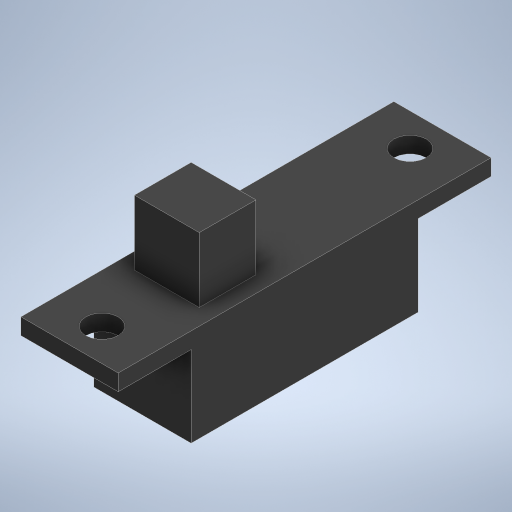
# Autodesk Inventor part: SlideSwitchj
Saved by Autodesk Inventor 2024.2 (Build 282272000, 272)
## iProperties
Created: 2024-05-04
Part Number: SlideSwitchj
Material: Generic
Document SubType Name: Modeling
Designer: ringl
Density: 1 g/cm^3
Appearance: Default(1)
Author: ringl
Autodesk Inventor part; units mm, degrees
ref_plane "YZ Plane" through (0, 0, 0) normal (1, 0, 0) x (0, 1, 0)
ref_plane "XZ Plane" through (0, 0, 0) normal (0, 1, 0) x (-1, 0, 0)
ref_plane "XY Plane" through (0, 0, 0) normal (0, 0, 1) x (1, 0, 0)
sketch "Sketch1" plane through (0, 0, 0) normal (0, 1, 0) x (-1, 0, 0)
  line L0 (0, 0) -> (6, 0)
  line L1 (6, 0) -> (6, -23)
  line L2 (6, -23) -> (0, -23)
  line L3 (0, -23) -> (0, 0)
  circle A0 centre (3, -2) radius 1
  circle A1 centre (3, -21) radius 1
  point P0 (3, 0)
  dimension "d0" = 6
  dimension "d1" = 23
  dimension "d2" = 2
  dimension "d3" = 2
  dimension "d4" = 19
  dimension "d5" = 2
  dimension "d6" = 3
  constraints: 8 end point, 2 centre point, 2 parallel, 1 horizontal, 1 midpoint, 1 perpendicular, 1 vertical alignment
  measures "d0" distance of L1.end L2.end
  measures "d1" distance of L0.end L1.end
  measures "d2" diameter of A0
  measures "d3" diameter of A1
  measures "d4" distance of A0.centre A1.centre
  measures "d5" distance of point (3, 0) A0.centre
  measures "d6" distance from line of L3 A1.centre
extrude "Extrusion1" add sketch "Sketch1" along normal blind 1
sketch "Sketch2" plane through (0, 0, 0) normal (0, -1, 0) x (1, 0, 0)
  line L0 (-6, -23) -> (-6, 0) projected
  line L1 (0, 0) -> (0, -23) projected
  line L2 (-6, -4.5) -> (0, -4.5)
  line L3 (0, -4.5) -> (0, -18.5)
  line L4 (0, -18.5) -> (-6, -18.5)
  line L5 (-6, -18.5) -> (-6, -4.5)
  line L6 (-6, 0) -> (0, 0) projected
  point P0 (-3, -18.5)
  dimension "d9" = 14
  dimension "d10" = 4.5
  constraints: 8 end point, 2 parallel, 2 point on line, 1 horizontal, 1 midpoint, 1 perpendicular
  measures "d9" distance from line of point (-3, -18.5) L2
  measures "d10" distance between parallel lines of L6 L2
extrude "Extrusion2" add sketch "Sketch2" along normal blind 5 contours L0 L2 L1 L4
sketch "Sketch3" plane through (0, 1, 0) normal (0, 1, 0) x (1, 0, 0)
  line L0 (-5, 6) -> (-1, 6)
  line L1 (-1, 6) -> (-1, 9.5)
  line L2 (-1, 9.5) -> (-5, 9.5)
  line L3 (-5, 9.5) -> (-5, 6)
  line L4 (-6, 23) -> (-6, 0) projected
  line L5 (-6, 0) -> (0, 0) projected
  dimension "d13" = 4
  dimension "d14" = 3.5
  dimension "d15" = 1
  dimension "d16" = 6
  constraints: 8 end point, 2 parallel, 1 horizontal, 1 perpendicular
  measures "d13" distance of L1.end L2.end
  measures "d14" distance of L0.end L1.end
  measures "d15" distance between parallel lines of L4 L3
  measures "d16" distance between parallel lines of L5 L0
extrude "Extrusion3" add sketch "Sketch3" along normal blind 4
body "Solid1"
